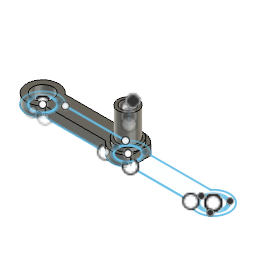
scissor end piece arm (Autodesk Fusion 360 design; units mm, degrees)
part number: 2025-11-19-16-47-52-691
part number: 2025-11-19-16-48-20-946
Autodesk Fusion 360 part; units mm, degrees
sketch "Sketch3" plane through (0, 0, 0) normal (0, 0, 1) x (1, 0, 0) in component "sciccor arm right size"
  line L0 (36.255, 10) -> (6.245, 10)
  line L1 (6.245, 0) -> (36.255, 0)
  line L2 (48.745, 0) -> (78.755, 0)
  line L3 (78.755, 10) -> (48.745, 10)
  arc A0 (78.755, 0) -> (78.755, 10) centre (85, 5) ccw
  arc A1 (48.745, 10) -> (36.255, 10) centre (42.5, 5) ccw
  arc A2 (36.255, 0) -> (48.745, 0) centre (42.5, 5) ccw
  arc A3 (6.245, 10) -> (6.245, 0) centre (0, 5) ccw
  circle A4 centre (0, 5) radius 5.0725
  circle A5 centre (42.5, 5) radius 5.0725
  circle A6 centre (85, 5) radius 5.0725
  line L4 (48.745, 0) -> (78.755, 0)
  line L5 (36.255, 10) -> (6.245, 10)
  circle A7 centre (85, 5) radius 5.0725
  circle A8 centre (42.5, 5) radius 5.0725
  line L6 (6.245, 0) -> (36.255, 0)
  circle A9 centre (0, 5) radius 5.0725
  line L7 (36.255, 10) -> (6.245, 10)
  line L8 (36.255, 10) -> (6.245, 10)
  circle A10 centre (85, 5) radius 5.0725
  circle A11 centre (85, 5) radius 5.0725
  circle A12 centre (42.5, 5) radius 5.0725
  circle A13 centre (42.5, 5) radius 5.0725
  circle A14 centre (0, 5) radius 5.0725
  circle A15 centre (0, 5) radius 5.0725
  circle A16 centre (85, 5) radius 5.0725
  circle A17 centre (85, 5) radius 5.0725
  circle A18 centre (85, 5) radius 5.0725
  circle A19 centre (85, 5) radius 5.0725
  circle A20 centre (42.5, 5) radius 5.0725
  circle A21 centre (42.5, 5) radius 5.0725
  circle A22 centre (42.5, 5) radius 5.0725
  circle A23 centre (42.5, 5) radius 5.0725
  circle A24 centre (0, 5) radius 5.0725
  circle A25 centre (0, 5) radius 5.0725
  circle A26 centre (0, 5) radius 5.0725
  circle A27 centre (0, 5) radius 5.0725
  arc A28 (48.745, 10) -> (36.255, 10) centre (42.5, 5) ccw
  line L9 (36.255, 10) -> (6.245, 10)
  arc A29 (6.245, 10) -> (6.245, 0) centre (0, 5) ccw
  line L10 (78.755, 10) -> (48.745, 10)
  line L11 (48.745, 0) -> (78.755, 0)
  arc A30 (78.755, 0) -> (78.755, 10) centre (85, 5) ccw
  arc A31 (36.255, 0) -> (48.745, 0) centre (42.5, 5) ccw
  line L12 (6.245, 0) -> (36.255, 0)
  circle A32 centre (85, 5) radius 6
  circle A33 centre (79, 5) radius 0.9275
  circle A34 centre (88.4216, 9.9287) radius 0.9275
  circle A35 centre (88.4216, 0.0713) radius 0.9275
  circle A36 centre (42.5, 5) radius 6
  circle A37 centre (0, 5) radius 6
  circle A38 centre (36.5, 5.0009) radius 0.9275
  circle A39 centre (45.9319, 9.9216) radius 0.9275
  circle A40 centre (45.9319, 0.0784) radius 0.9275
  circle A41 centre (-6, 5) radius 0.9275
  circle A42 centre (3.2447, 10.047) radius 0.9275
  circle A43 centre (3.2447, -0.047) radius 0.9275
  point P0 (85, 5)
  point P1 (36.255, 0)
  point P2 (85, 5)
  dimension "d25" = 16
  dimension "d27" = 16
  dimension "d30" = 16
  dimension "d34" = 10.145
  dimension "d35" = 10.145
  dimension "d36" = 10.145
  dimension "d37" = 10.145
  dimension "d38" = 10.145
  dimension "d39" = 10.145
  dimension "d40" = 10.145
  dimension "d41" = 10.145
  dimension "d42" = 10.145
  dimension "d43" = 10.145
  dimension "d44" = 10.145
  dimension "d45" = 10.145
  dimension "d46" = 16
  dimension "d47" = 16
  dimension "d48" = 16
  dimension "d49" = 10.145
  dimension "d50" = 10.145
  dimension "d51" = 10.145
  dimension "d52" = 10.145
  dimension "d53" = 10.145
  dimension "d54" = 10.145
  dimension "d55" = 10.145
  dimension "d56" = 10.145
  dimension "d57" = 10.145
  dimension "d58" = 10.145
  dimension "d59" = 10.145
  dimension "d60" = 10.145
  dimension "d61" = 12
  dimension "d62" = 12
  dimension "d63" = 12
  constraint coincident P1 A1
  constraint concentric A1 A2
  constraint concentric A3 A4
  constraint concentric A2 A5
  constraint concentric A0 A6
  constraint coincident P1 A28
  constraint concentric A28 A31
  constraint concentric A25 A29
  constraint concentric A23 A31
  constraint concentric A17 A30
  constraint concentric A7 A32
  constraint coincident A32 A33.centre
  constraint tangent A10 A33
  constraint coincident A32 A34.centre
  constraint tangent A7 A34
  constraint coincident A32 A35.centre
  constraint tangent A17 A35
  constraint concentric A8 A36
  constraint concentric A3 A37
  constraint coincident A36 A38.centre
  constraint tangent A23 A38
  constraint coincident A36 A39.centre
  constraint tangent A8 A39
  constraint coincident A36 A40.centre
  constraint tangent A5 A40
  constraint coincident A37 A41.centre
  constraint tangent A9 A41
  constraint coincident A37 A42.centre
  constraint tangent A15 A42
  constraint coincident A37 A43.centre
  constraint tangent A14 A43
  measures "d25" diameter of A1
  measures "d27" diameter of A0
  measures "d30" diameter of A3
  measures "d34" diameter of A4
  measures "d35" diameter of A5
  measures "d36" diameter of A6
  measures "d37" diameter of A9
  measures "d38" diameter of A8
  measures "d39" diameter of A7
  measures "d40" diameter of A15
  measures "d41" diameter of A13
  measures "d42" diameter of A11
  measures "d43" diameter of A14
  measures "d44" diameter of A12
  measures "d45" diameter of A10
  measures "d46" diameter of A28
  measures "d47" diameter of A30
  measures "d48" diameter of A29
  measures "d49" diameter of A25
  measures "d50" diameter of A23
  measures "d51" diameter of A17
  measures "d52" diameter of A26
  measures "d53" diameter of A20
  measures "d54" diameter of A18
  measures "d55" diameter of A27
  measures "d56" diameter of A21
  measures "d57" diameter of A19
  measures "d58" diameter of A24
  measures "d59" diameter of A22
  measures "d60" diameter of A16
  measures "d61" diameter of A32
  measures "d62" diameter of A36
  measures "d63" diameter of A37
extrude "Extrude1" add sketch "Sketch3" along normal blind 5 contours L0 L1 L2 L3 A0 A1 A2 A3 L4 L5 L6 L7 L8 A28 L9 A29 L10 L11 A30 A31 L12 | A4 A9 A14 A15 A24 A25 A26 A27 A37 A42 A43 | A4 A9 A14 A15 A24 A25 A26 A27 A37 A41 A42 | A37 A42 | A4 A9 A14 A15 A24 A25 A26 A27 A37 A41 A43 | A37 A43 | A37 A41 | A37 A42 | A37 A43 | A37 A41 | A5 A8 A12 A13 A20 A21 A22 A23 A36 A39 A40 | A5 A8 A12 A13 A20 A21 A22 A23 A36 A38 A39 | A36 A39 | A5 A8 A12 A13 A20 A21 A22 A23 A36 A38 A40 | A36 A40 | A36 A38 | A36 A39 | A36 A40 | A36 A38 | A6 A7 A10 A11 A16 A17 A18 A19 A32 A34 A35 | A6 A7 A10 A11 A16 A17 A18 A19 A32 A33 A34 | A32 A34 | A6 A7 A10 A11 A16 A17 A18 A19 A32 A33 A35 | A32 A35 | A32 A33 | A32 A34 | A32 A35 | A32 A33 makes body 1
ref_plane "WorkPlane1" through (94, 0, 0) normal (1, 0, 0) x (0, 1, 0)
sketch "Sketch1" plane through (94, 0, 0) normal (1, 0, 0) x (0, 1, 0)
  line L0 (-4.1622, 5.4388) -> (14.0327, 5.4388)
  line L1 (14.0327, 5.4388) -> (14.0327, -0.333)
  line L2 (14.0327, -0.333) -> (-4.1622, -0.333)
  line L3 (-4.1622, -0.333) -> (-4.1622, 5.4388)
  constraint horizontal L0
  constraint vertical L1
  constraint horizontal L2
  constraint vertical L3
extrude "Extrude2" cut sketch "Sketch1" against normal blind 45 bodies 1
sketch "Sketch2" plane through (0, 0, 5) normal (0, 0, 1) x (-1, 0, 0)
  line L0 (-49, 0) -> (-49, -10)
  line L1 (-49, -10) -> (-48.745, -10)
  arc A0 (-48.745, -10) -> (-36.255, -10) centre (-42.5, -5) ccw
  line L2 (-36.255, -10) -> (-6.245, -10)
  arc A1 (-6.245, -10) -> (-6.245, 0) centre (0, -5) ccw
  line L3 (-6.245, 0) -> (-36.255, 0)
  arc A2 (-36.255, 0) -> (-48.745, 0) centre (-42.5, -5) ccw
  line L4 (-48.745, 0) -> (-49, 0)
  circle A3 centre (-42.5, -5) radius 5.0725
  circle A4 centre (0, -5) radius 5.0725
  circle A5 centre (-42.5, -5) radius 6.2628
  constraint concentric A0 A5
extrude "Extrude3" add sketch "Sketch2" along normal blind 2 separate body contours A3 | A5 makes body 2
sketch "Sketch3 (2)" plane through (0, 0, 7) normal (0, 0, 1) x (-1, 0, 0)
  circle A0 centre (-42.5, -5) radius 6.2628
  circle A1 centre (-42.5, -5) radius 5
  dimension "d73" = 10
  constraint concentric A0 A1
  measures "d73" diameter of A1
extrude "Extrude4" add sketch "Sketch3 (2)" along normal blind 6 contours A1 bodies 2
sketch "Sketch8" plane through (0, 0, 0) normal (0, 0, 1) x (1, 0, 0)
  circle A0 centre (42.4473, 5.0398) radius 3.5
  dimension "d90" = 7
  measures "d90" diameter of A0
extrude "Extrude5" cut sketch "Sketch8" along normal blind 13 bodies 2
ref_plane "WorkPlane3" through (43, 0, 0) normal (1, 0, 0) x (0, 1, 0)
sketch "Sketch6" plane through (43, 0, 0) normal (1, 0, 0) x (0, 1, 0)
  spline S0 degree 5 poles (5, 13) (4.9316, 13.0722) (4.8094, 13.2327) (4.67, 13.5216) (4.5725, 14.0041) (4.5987, 14.7692) (4.7688, 15.6883) (5.0688, 16.74) (5.4689, 17.8804) (5.9208, 19.0405) (6.3658, 20.1371) (6.7412, 21.0814) (6.9866, 21.7885) (7.0505, 22.1858) (6.8986, 22.2261) (6.5169, 21.891) (6.0251, 21.3207) (5.5526, 20.7251) (5.1918, 20.254) (5, 20) knots 0 0 0 0 0 0 0.066667 0.133333 0.2 0.266667 0.333333 0.4 0.466667 0.533333 0.6 0.666667 0.733333 0.8 0.866667 0.933333 1 1 1 1 1 1
  point P0 (5, 16.4583)
  point P1 (7, 22)
sketch "Sketch7" plane through (0, 0, 13) normal (0, 0, 1) x (-1, 0, 0)
  circle A0 centre (-42.5, -5) radius 5
  circle A1 centre (-42.377, -5) radius 3.652
  circle A2 centre (-42.4473, -5.0398) radius 3.5
extrude "Extrude6" add 1 faces at (46.8379, 3.9297, 13) along direction (0, 0, 1) blind 8 on bodies 2 bodies 2
component "sciccor arm right size" placed x (1, 0, 0) y (0, 1, 0) z (0, 0, 1) at (0, 0, 0)
